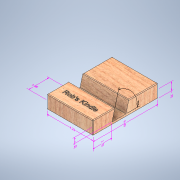
# Autodesk Inventor part: robsKindleStand
Saved by Autodesk Inventor 2020.2 (Build 242310000, 310)
## iProperties
Created: 2020-01-24
Part Number: robsKindleStand
Material: Wood (Birch)
Document SubType Name: Modeling
Designer: steele
Density: 0.55 g/cm^3
Appearance: Birch - Natural Polished
Author: steele
Autodesk Inventor part; units mm, degrees
ref_plane "YZ Plane" through (0, 0, 0) normal (1, 0, 0) x (0, 1, 0)
ref_plane "XZ Plane" through (0, 0, 0) normal (0, 1, 0) x (-1, 0, 0)
ref_plane "XY Plane" through (0, 0, 0) normal (0, 0, 1) x (1, 0, 0)
sketch "Sketch2" plane through (0, 0, 0) normal (0, 1, 0) x (-1, 0, 0)
  line L0 (53.975, 76.2) -> (-53.975, 76.2)
  line L1 (-53.975, 76.2) -> (-53.975, -76.2)
  line L2 (-53.975, -76.2) -> (53.975, -76.2)
  line L3 (53.975, -76.2) -> (53.975, 76.2)
  line L4 (53.975, 76.2) -> (-53.975, -76.2) construction
  line L5 (-53.975, 76.2) -> (53.975, -76.2) construction
  point P0 (0, 0)
  dimension "d0" = 107.95
  dimension "d1" = 152.4
  constraints: 12 end point, 2 midpoint, 2 parallel, 1 horizontal, 1 perpendicular
  measures "d0" distance of L0.start L0.end
  measures "d1" distance of L1.end L0.end
extrude "Extrusion1" add sketch "Sketch2" along normal blind 31.75
sketch "Sketch4" plane through (53.975, 0, 76.2) normal (1, 0, 0) x (0, 0, -1)
  line L0 (0, 31.75) -> (152.4, 31.75) projected
  line L1 (84.1259, 31.75) -> (77.32, 6.35)
  line L2 (77.32, 6.35) -> (44.45, 6.35)
  line L3 (44.45, 6.35) -> (51.2559, 31.75)
  line L4 (84.1259, 31.75) -> (51.2559, 31.75)
  line L5 (0, 0) -> (0, 31.75) projected
  point P0 (76.2, 0)
  point P1 (73.5162, 12.7)
  dimension "d27" = 25.4
  dimension "d28" = 44.45
  dimension "d29" = 75
  dimension "d46" = 31.75
  constraints: 8 end point, 2 parallel, 1 horizontal, 3 other
  measures "d28" distance from line of L5 L2.end
  measures "d29" angle of L3 L2
  measures "d46" distance between parallel lines of L1 L3
extrude "Extrusion3" cut sketch "Sketch4" against normal through all
sketch "Sketch6" plane through (0, 31.75, 0) normal (0, 1, 0) x (1, 0, 0)
  line L0 (-53.975, -24.9441) -> (-53.975, -76.2) construction
  line L1 (-53.975, -50.8) -> (53.975, -50.8) construction
  line L2 (53.975, -76.2) -> (53.975, -24.9441) construction
  line L3 (-53.975, -76.2) -> (53.975, -76.2) construction
  line L4 (-38.5027, -55.88) -> (-38.5027, -45.72)
  line L5 (-38.5027, -45.72) -> (-33.9957, -45.72)
  spline S0 degree 2 poles (-33.9957, -45.72) (-32.6406, -45.72) (-31.2234, -46.2698) (-30.3793, -47.656) (-30.3793, -48.4923) knots 0 0 0 1 2 3 3 3
  spline S1 degree 2 poles (-30.3793, -48.4923) (-30.3793, -49.5765) (-31.781, -51.0555) (-33.2368, -51.2569) knots 0 0 0 1 2 2 2
  spline S2 degree 2 poles (-33.2368, -51.2569) (-32.7102, -51.5124) (-32.4315, -51.7602) knots 0 0 0 1 1 1
  spline S3 degree 2 poles (-32.4315, -51.7602) (-31.8429, -52.3023) (-31.3163, -53.1154) knots 0 0 0 1 1 1
  line L6 (-31.3163, -53.1154) -> (-29.5585, -55.88)
  line L7 (-29.5585, -55.88) -> (-31.2389, -55.88)
  line L8 (-31.2389, -55.88) -> (-32.5863, -53.7659)
  spline S4 degree 2 poles (-32.5863, -53.7659) (-33.1749, -52.8521) (-33.9338, -51.8841) (-34.5378, -51.4892) (-34.8476, -51.4118) knots 0 0 0 1 2 3 3 3
  spline S5 degree 2 poles (-34.8476, -51.4118) (-35.0799, -51.3653) (-35.5987, -51.3653) knots 0 0 0 1 1 1
  line L9 (-35.5987, -51.3653) -> (-37.1552, -51.3653)
  line L10 (-37.1552, -51.3653) -> (-37.1552, -55.88)
  line L11 (-37.1552, -55.88) -> (-38.5027, -55.88)
  line L12 (-37.1552, -50.2037) -> (-34.2668, -50.2037)
  spline S6 degree 2 poles (-34.2668, -50.2037) (-33.3452, -50.2037) (-32.3076, -49.8243) (-31.7655, -48.9802) (-31.7655, -48.4923) knots 0 0 0 1 2 3 3 3
  spline S7 degree 2 poles (-31.7655, -48.4923) (-31.7655, -47.7721) (-32.8109, -46.8429) (-33.9415, -46.8429) knots 0 0 0 1 2 2 2
  line L13 (-33.9415, -46.8429) -> (-37.1552, -46.8429)
  line L14 (-37.1552, -46.8429) -> (-37.1552, -50.2037)
  spline S8 degree 2 poles (-28.8925, -52.1939) (-28.8925, -50.1573) (-27.7541, -49.1738) knots 0 0 0 1 1 1
  spline S9 degree 2 poles (-27.7541, -49.1738) (-26.8094, -48.3529) (-25.4465, -48.3529) knots 0 0 0 1 1 1
  spline S10 degree 2 poles (-25.4465, -48.3529) (-23.9287, -48.3529) (-22.0004, -50.3431) (-22.0004, -52.0932) knots 0 0 0 1 2 2 2
  spline S11 degree 2 poles (-22.0004, -52.0932) (-22.0004, -53.5104) (-22.8523, -55.1443) (-24.4785, -56.0426) (-25.4465, -56.0426) knots 0 0 0 1 2 3 3 3
  spline S12 degree 2 poles (-25.4465, -56.0426) (-26.9875, -56.0426) (-28.8925, -54.0602) (-28.8925, -52.1939) knots 0 0 0 1 2 2 2
  spline S13 degree 2 poles (-27.607, -52.2016) (-27.607, -53.611) (-26.3757, -55.0204) (-25.4465, -55.0204) knots 0 0 0 1 2 2 2
  spline S14 degree 2 poles (-25.4465, -55.0204) (-24.5172, -55.0204) (-23.2859, -53.6033) (-23.2859, -52.1552) knots 0 0 0 1 2 2 2
  spline S15 degree 2 poles (-23.2859, -52.1552) (-23.2859, -50.7923) (-24.5249, -49.3829) (-25.4465, -49.3829) knots 0 0 0 1 2 2 2
  spline S16 degree 2 poles (-25.4465, -49.3829) (-26.3757, -49.3829) (-27.607, -50.7845) (-27.607, -52.2016) knots 0 0 0 1 2 2 2
  line L15 (-19.3907, -55.88) -> (-20.5446, -55.88)
  line L16 (-20.5446, -55.88) -> (-20.5446, -45.72)
  line L17 (-20.5446, -45.72) -> (-19.2978, -45.72)
  line L18 (-19.2978, -45.72) -> (-19.2978, -49.3441)
  spline S17 degree 2 poles (-19.2978, -49.3441) (-18.5079, -48.3529) (-17.2844, -48.3529) knots 0 0 0 1 1 1
  spline S18 degree 2 poles (-17.2844, -48.3529) (-16.6029, -48.3529) (-15.3871, -48.9027) (-14.605, -49.894) (-14.1636, -51.2879) (-14.1636, -52.0855) knots 0 0 0 1 2 3 4 4 4
  spline S19 degree 2 poles (-14.1636, -52.0855) (-14.1636, -53.975) (-16.0376, -56.0426) (-17.3463, -56.0426) knots 0 0 0 1 2 2 2
  spline S20 degree 2 poles (-17.3463, -56.0426) (-18.6473, -56.0426) (-19.3907, -54.9585) knots 0 0 0 1 1 1
  line L19 (-19.3907, -54.9585) -> (-19.3907, -55.88)
  spline S21 degree 2 poles (-19.4062, -52.1397) (-19.4062, -53.4639) (-19.05, -54.0602) knots 0 0 0 1 1 1
  spline S22 degree 2 poles (-19.05, -54.0602) (-18.4615, -55.0204) (-17.4548, -55.0204) knots 0 0 0 1 1 1
  spline S23 degree 2 poles (-17.4548, -55.0204) (-16.6416, -55.0204) (-15.4491, -53.5955) (-15.4491, -52.1939) knots 0 0 0 1 2 2 2
  spline S24 degree 2 poles (-15.4491, -52.1939) (-15.4491, -50.7458) (-16.5874, -49.3751) (-17.4006, -49.3751) knots 0 0 0 1 2 2 2
  spline S25 degree 2 poles (-17.4006, -49.3751) (-18.2137, -49.3751) (-19.4062, -50.8) (-19.4062, -52.1397) knots 0 0 0 1 2 2 2
  line L20 (-12.6381, -49.3209) -> (-12.9556, -47.4237)
  line L21 (-12.9556, -47.4237) -> (-12.9556, -45.72)
  line L22 (-12.9556, -45.72) -> (-11.5384, -45.72)
  line L23 (-11.5384, -45.72) -> (-11.5384, -47.4237)
  line L24 (-11.5384, -47.4237) -> (-11.8714, -49.3209)
  line L25 (-11.8714, -49.3209) -> (-12.6381, -49.3209)
  line L26 (-10.4388, -53.6807) -> (-9.2075, -53.4871)
  spline S26 degree 2 poles (-9.2075, -53.4871) (-9.1068, -54.2305) (-8.1543, -55.0204) (-7.2948, -55.0204) knots 0 0 0 1 2 2 2
  spline S27 degree 2 poles (-7.2948, -55.0204) (-6.4352, -55.0204) (-5.5988, -54.3157) (-5.5988, -53.8434) knots 0 0 0 1 2 2 2
  spline S28 degree 2 poles (-5.5988, -53.8434) (-5.5988, -53.4252) (-5.9706, -53.1774) knots 0 0 0 1 1 1
  spline S29 degree 2 poles (-5.9706, -53.1774) (-6.2261, -53.0148) (-7.2483, -52.7592) knots 0 0 0 1 1 1
  spline S30 degree 2 poles (-7.2483, -52.7592) (-8.619, -52.4107) (-9.6799, -51.9074) (-10.2297, -51.0091) (-10.2297, -50.4748) knots 0 0 0 1 2 3 3 3
  spline S31 degree 2 poles (-10.2297, -50.4748) (-10.2297, -49.9791) (-9.7806, -49.1428) (-9.3934, -48.864) knots 0 0 0 1 2 2 2
  spline S32 degree 2 poles (-9.3934, -48.864) (-9.0991, -48.6472) (-8.0924, -48.3529) (-7.5116, -48.3529) knots 0 0 0 1 2 2 2
  spline S33 degree 2 poles (-7.5116, -48.3529) (-6.6443, -48.3529) (-5.3356, -48.8563) (-4.7083, -49.7081) (-4.5921, -50.4205) knots 0 0 0 1 2 3 3 3
  line L27 (-4.5921, -50.4205) -> (-5.8157, -50.5832)
  spline S34 degree 2 poles (-5.8157, -50.5832) (-5.9009, -50.0101) (-6.6985, -49.3751) (-7.4264, -49.3751) knots 0 0 0 1 2 2 2
  spline S35 degree 2 poles (-7.4264, -49.3751) (-8.286, -49.3751) (-9.0216, -49.9482) (-9.0216, -50.3276) knots 0 0 0 1 2 2 2
  spline S36 degree 2 poles (-9.0216, -50.3276) (-9.0216, -50.5677) (-8.8668, -50.7613) knots 0 0 0 1 1 1
  spline S37 degree 2 poles (-8.8668, -50.7613) (-8.7196, -50.9626) (-8.3866, -51.0943) knots 0 0 0 1 1 1
  spline S38 degree 2 poles (-8.3866, -51.0943) (-8.2008, -51.164) (-7.287, -51.4195) knots 0 0 0 1 1 1
  spline S39 degree 2 poles (-7.287, -51.4195) (-5.9628, -51.768) (-4.9096, -52.2171) (-4.3134, -53.0767) (-4.3134, -53.7195) knots 0 0 0 1 2 3 3 3
  spline S40 degree 2 poles (-4.3134, -53.7195) (-4.3134, -54.339) (-5.0413, -55.4386) (-6.4197, -56.0426) (-7.287, -56.0426) knots 0 0 0 1 2 3 3 3
  spline S41 degree 2 poles (-7.287, -56.0426) (-8.7196, -56.0426) (-10.2297, -54.8501) (-10.4388, -53.6807) knots 0 0 0 1 2 2 2
  line L28 (1.208, -55.88) -> (1.208, -45.72)
  line L29 (1.208, -45.72) -> (2.5555, -45.72)
  line L30 (2.5555, -45.72) -> (2.5555, -50.7535)
  line L31 (2.5555, -50.7535) -> (7.6045, -45.72)
  line L32 (7.6045, -45.72) -> (9.4243, -45.72)
  line L33 (9.4243, -45.72) -> (5.1652, -49.8398)
  line L34 (5.1652, -49.8398) -> (9.6102, -55.88)
  line L35 (9.6102, -55.88) -> (7.8368, -55.88)
  line L36 (7.8368, -55.88) -> (4.2204, -50.7458)
  line L37 (4.2204, -50.7458) -> (2.5555, -52.3565)
  line L38 (2.5555, -52.3565) -> (2.5555, -55.88)
  line L39 (2.5555, -55.88) -> (1.208, -55.88)
  line L40 (10.5859, -55.88) -> (10.5859, -48.5155)
  line L41 (10.5859, -48.5155) -> (11.8327, -48.5155)
  line L42 (11.8327, -48.5155) -> (11.8327, -55.88)
  line L43 (11.8327, -55.88) -> (10.5859, -55.88)
  line L44 (10.5859, -47.1526) -> (10.5859, -45.72)
  line L45 (10.5859, -45.72) -> (11.8327, -45.72)
  line L46 (11.8327, -45.72) -> (11.8327, -47.1526)
  line L47 (11.8327, -47.1526) -> (10.5859, -47.1526)
  line L48 (13.7299, -55.88) -> (13.7299, -48.5155)
  line L49 (13.7299, -48.5155) -> (14.8528, -48.5155)
  line L50 (14.8528, -48.5155) -> (14.8528, -49.561)
  spline S42 degree 2 poles (14.8528, -49.561) (15.6659, -48.3529) (17.1915, -48.3529) knots 0 0 0 1 1 1
  spline S43 degree 2 poles (17.1915, -48.3529) (17.8574, -48.3529) (18.9726, -48.833) (19.5301, -49.6074) (19.6385, -50.1418) knots 0 0 0 1 2 3 3 3
  spline S44 degree 2 poles (19.6385, -50.1418) (19.7082, -50.4902) (19.7082, -51.3576) knots 0 0 0 1 1 1
  line L51 (19.7082, -51.3576) -> (19.7082, -55.88)
  line L52 (19.7082, -55.88) -> (18.4615, -55.88)
  line L53 (18.4615, -55.88) -> (18.4615, -51.404)
  spline S45 degree 2 poles (18.4615, -51.404) (18.4615, -50.6451) (18.1672, -49.8862) (17.4315, -49.4371) (16.9282, -49.4371) knots 0 0 0 1 2 3 3 3
  spline S46 degree 2 poles (16.9282, -49.4371) (16.1305, -49.4371) (14.9767, -50.4515) (14.9767, -51.8609) knots 0 0 0 1 2 2 2
  line L54 (14.9767, -51.8609) -> (14.9767, -55.88)
  line L55 (14.9767, -55.88) -> (13.7299, -55.88)
  line L56 (26.399, -55.88) -> (26.399, -54.9507)
  spline S47 degree 2 poles (26.399, -54.9507) (25.702, -56.0426) (24.3391, -56.0426) knots 0 0 0 1 1 1
  spline S48 degree 2 poles (24.3391, -56.0426) (23.4563, -56.0426) (21.9849, -55.0746) (21.1718, -53.3323) (21.1718, -52.2016) knots 0 0 0 1 2 3 3 3
  spline S49 degree 2 poles (21.1718, -52.2016) (21.1718, -51.102) (21.9075, -49.3054) (23.3711, -48.3529) (24.2771, -48.3529) knots 0 0 0 1 2 3 3 3
  spline S50 degree 2 poles (24.2771, -48.3529) (24.9431, -48.3529) (25.9808, -48.9105) (26.306, -49.3596) knots 0 0 0 1 2 2 2
  line L57 (26.306, -49.3596) -> (26.306, -45.72)
  line L58 (26.306, -45.72) -> (27.5528, -45.72)
  line L59 (27.5528, -45.72) -> (27.5528, -55.88)
  line L60 (27.5528, -55.88) -> (26.399, -55.88)
  spline S51 degree 2 poles (22.4573, -52.2016) (22.4573, -53.6188) (23.6499, -55.0204) (24.463, -55.0204) knots 0 0 0 1 2 2 2
  spline S52 degree 2 poles (24.463, -55.0204) (25.2761, -55.0204) (26.4222, -53.6807) (26.4222, -52.3101) knots 0 0 0 1 2 2 2
  spline S53 degree 2 poles (26.4222, -52.3101) (26.4222, -50.8) (25.2606, -49.3829) (24.4088, -49.3829) knots 0 0 0 1 2 2 2
  spline S54 degree 2 poles (24.4088, -49.3829) (23.5724, -49.3829) (22.4573, -50.7458) (22.4573, -52.2016) knots 0 0 0 1 2 2 2
  line L61 (29.481, -55.88) -> (29.481, -45.72)
  line L62 (29.481, -45.72) -> (30.7278, -45.72)
  line L63 (30.7278, -45.72) -> (30.7278, -55.88)
  line L64 (30.7278, -55.88) -> (29.481, -55.88)
  line L65 (37.6973, -53.5026) -> (38.9905, -53.6652)
  spline S55 degree 2 poles (38.9905, -53.6652) (38.6808, -54.7959) (37.0313, -56.0426) (35.7536, -56.0426) knots 0 0 0 1 2 2 2
  spline S56 degree 2 poles (35.7536, -56.0426) (34.1351, -56.0426) (32.2456, -54.0524) (32.2456, -52.2636) knots 0 0 0 1 2 2 2
  spline S57 degree 2 poles (32.2456, -52.2636) (32.2456, -50.4051) (34.1584, -48.3529) (35.6839, -48.3529) knots 0 0 0 1 2 2 2
  spline S58 degree 2 poles (35.6839, -48.3529) (37.1552, -48.3529) (39.0293, -50.3663) (39.0293, -52.1862) knots 0 0 0 1 2 2 2
  spline S59 degree 2 poles (39.0293, -52.1862) (39.0293, -52.2946) (39.0215, -52.5191) knots 0 0 0 1 1 1
  line L66 (39.0215, -52.5191) -> (33.5311, -52.5191)
  spline S60 degree 2 poles (33.5311, -52.5191) (33.6008, -53.7349) (34.8321, -55.0204) (35.7536, -55.0204) knots 0 0 0 1 2 2 2
  spline S61 degree 2 poles (35.7536, -55.0204) (36.4428, -55.0204) (37.4108, -54.2925) (37.6973, -53.5026) knots 0 0 0 1 2 2 2
  line L67 (33.6008, -51.497) -> (37.7128, -51.497)
  spline S62 degree 2 poles (37.7128, -51.497) (37.6276, -50.5677) (37.2404, -50.0953) knots 0 0 0 1 1 1
  spline S63 degree 2 poles (37.2404, -50.0953) (36.6441, -49.3751) (35.6916, -49.3751) knots 0 0 0 1 1 1
  spline S64 degree 2 poles (35.6916, -49.3751) (34.8321, -49.3751) (33.6627, -50.529) (33.6008, -51.497) knots 0 0 0 1 2 2 2
  point P0 (0, 0)
  dimension "d50" = 25.4
  constraints: 2 end point, 2 horizontal, 2 point on line
  measures "d50" distance between parallel lines of L1 L3
extrude "Extrusion4" cut sketch "Sketch6" against normal blind 2.54
fillet "Fillet1" radius 1.5875 16 edges at (0, 31.75, -7.9259) (0, 31.75, 24.9441) (0, 31.75, 76.2) (0, 31.75, -76.2) (-53.975, 31.75, -42.063) (53.975, 31.75, -42.063) (53.975, 31.75, 50.572) (-53.975, 31.75, 50.572) (0, 0, 76.2) (-53.975, 15.875, 76.2) (53.975, 15.875, 76.2) (53.975, 0, 0) (53.975, 15.875, -76.2) (0, 0, -76.2) (-53.975, 15.875, -76.2) (-53.975, 0, 0)
body "Solid1"
